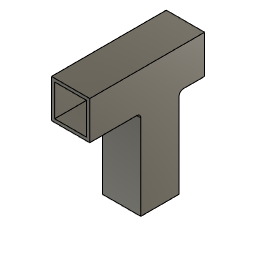
suporte+motor+90º (Autodesk Fusion 360 design; units mm, degrees)
Autodesk Fusion 360 part; units mm, degrees
form "Forma1" [no effect]
box "Primitiva de caixa1" add length 30 width 30 height 70 placed x (0, -1, 0) y (1, 0, 0) z (0, 0, 1) at (-30, 0, 0)
box "Primitiva de caixa2" add length 30 width 30 height -70 placed x (0, 0, 1) y (1, 0, 0) z (0, 1, 0) at (-30, 0, 70)
box "Primitiva de caixa3" add length 30 width 30 height 20 placed x (0, 0, -1) y (-1, 0, 0) z (0, 1, 0) at (0, 0, 100)
shell "Casca1" thickness 5 removed faces 0 bodies 1
box "Primitiva de caixa4" cut length 25 width 25 height -85 placed x (0, 0, 1) y (-1, 0, 0) z (0, -1, 0) at (-2.5, -70, 72.5)
box "Primitiva de caixa5" cut length 10 width 10 height -6 placed x (0, 1, 0) y (1, 0, 0) z (0, 0, -1) at (-20, 5, 70)
cylinder "Cilindro primitivo1" cut diameter 10 height -63 placed x (0, 1, 0) y (1, 0, 0) z (0, 0, -1) at (-15, -15, 0)
fillet "Arredondamento1" radius 3 1 edges at (-15, -30, 70)
fillet "Arredondamento2" radius 3.5 1 edges at (-15, 0, 70)
